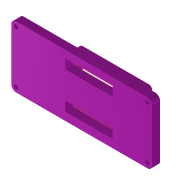
# Autodesk Inventor part: ESP32ParasiteMicroscope_base_v0
Saved by Autodesk Inventor 2022 (Build 260153000, 153)
## iProperties
Created: 2022-02-02
Part Number: ESP32ParasiteMicroscope_base_v0
Material: Generisch
Document SubType Name: Modeling
Designer: diederichbenedict
Density: 1 g/cm^3
Appearance: Glatt - Violett
Author: diederichbenedict
Autodesk Inventor part; units mm, degrees
ref_plane "YZ Plane" through (0, 0, 0) normal (1, 0, 0) x (0, 1, 0)
ref_plane "XZ Plane" through (0, 0, 0) normal (0, 1, 0) x (-1, 0, 0)
ref_plane "XY Plane" through (0, 0, 0) normal (0, 0, 1) x (1, 0, 0)
ref_plane "Arbeitsebene1" through (0, 0, 4) normal (0, 0, 1) x (1, 0, 0)
sketch "Skizze1" plane through (0, 0, 4) normal (0, 0, 1) x (1, 0, 0)
  arc A0 (-20, -12.5) -> (-19, -13.5) centre (-19, -12.5) ccw construction
  line L0 (-19, -13.5) -> (19, -13.5) construction
  arc A1 (19, -13.5) -> (20, -12.5) centre (19, -12.5) ccw construction
  line L1 (20, -12.5) -> (20, 12.5) construction
  arc A2 (20, 12.5) -> (19, 13.5) centre (19, 12.5) ccw construction
  line L2 (19, 13.5) -> (-19, 13.5) construction
  arc A3 (-19, 13.5) -> (-20, 12.5) centre (-19, 12.5) ccw construction
  line L3 (-20, 12.5) -> (-20, -12.5) construction
  line L4 (26, 12.5) -> (26, -12.5) construction
  arc A4 (19, -19.5) -> (26, -12.5) centre (19, -12.5) ccw construction
  line L5 (19, -19.5) -> (-19, -19.5) construction
  arc A5 (-26, -12.5) -> (-19, -19.5) centre (-19, -12.5) ccw construction
  line L6 (-26, -12.5) -> (-26, 12.5) construction
  arc A6 (-19, 19.5) -> (-26, 12.5) centre (-19, 12.5) ccw construction
  line L7 (-19, 19.5) -> (19, 19.5) construction
  arc A7 (26, 12.5) -> (19, 19.5) centre (19, 12.5) ccw construction
  line L8 (-24, 19.5) -> (19, 19.5)
  line L9 (19, 19.5) -> (19, -19.4749)
  line L10 (19, -19.4749) -> (-24, -19.4749)
  line L11 (-24, -19.4749) -> (-24, 19.5)
  line L12 (2.5735, 11.7657) -> (-15.3535, 11.7657) construction
  line L13 (2.5735, 13.7657) -> (-15.3535, 13.7657)
  line L14 (-15.3535, 9.7657) -> (2.5735, 9.7657)
  arc A8 (2.5735, 9.7657) -> (2.5735, 13.7657) centre (2.5735, 11.7657) ccw
  arc A9 (-15.3535, 13.7657) -> (-15.3535, 9.7657) centre (-15.3535, 11.7657) ccw
  line L15 (2.4395, -11.3613) -> (-15.3535, -11.3613) construction
  line L16 (2.4395, -9.3613) -> (-15.3535, -9.3613)
  line L17 (-15.3535, -13.3613) -> (2.4395, -13.3613)
  arc A10 (2.4395, -13.3613) -> (2.4395, -9.3613) centre (2.4395, -11.3613) ccw
  arc A11 (-15.3535, -9.3613) -> (-15.3535, -13.3613) centre (-15.3535, -11.3613) ccw
  circle A12 centre (-8.6034, 0.0126) radius 1.0539 construction
  line L18 (26.7026, 12.7126) -> (26.7026, -12.6874) construction
  line L19 (-48.7974, 12.7126) -> (26.7026, 12.7126) construction
  line L20 (-48.7974, -12.6874) -> (-48.7974, 12.7126) construction
  line L21 (26.7026, -12.6874) -> (-48.7974, -12.6874) construction
  line L22 (33.4901, -16.4749) -> (33.4901, 19.5) construction
  line L23 (30.4901, 19.5) -> (-52.5848, 19.5) construction
  line L24 (-55.5848, 19.5) -> (-55.5848, -16.4749) construction
  line L25 (-52.5848, -19.4749) -> (33.4901, -19.4749) construction
  line L26 (33.4901, 19.5) -> (19, 19.5)
  line L27 (19, 19.5) -> (19, -19.4749)
  line L28 (19, -19.4749) -> (30.4901, -19.4749)
  line L29 (33.4901, -19.4749) -> (33.4901, 16.5)
  line L30 (-24, 19.5) -> (-55.5848, 19.5)
  line L31 (-55.5848, 16.5) -> (-55.5848, -19.4749)
  line L32 (-55.5848, -19.4749) -> (-24, -19.4749)
  line L33 (-24, -19.4749) -> (-24, 19.5)
  arc A13 (-55.5848, -16.4749) -> (-52.5848, -19.4749) centre (-52.5848, -16.4749) ccw
  arc A14 (-52.5848, 19.5) -> (-55.5848, 16.5) centre (-52.5848, 16.5) ccw
  arc A15 (33.4901, 16.5) -> (30.4901, 19.5) centre (30.4901, 16.5) ccw
  arc A16 (30.4901, -19.4749) -> (33.4901, -16.4749) centre (30.4901, -16.4749) ccw
  line L34 (8.61, 8.7657) -> (-21.39, 8.7657)
  line L35 (-21.39, 8.7657) -> (-21.39, 14.7657)
  line L36 (-21.39, 14.7657) -> (8.61, 14.7657)
  line L37 (8.61, 14.7657) -> (8.61, 8.7657)
  line L38 (8.61, 8.7657) -> (-21.39, 14.7657) construction
  line L39 (-21.39, 8.7657) -> (8.61, 14.7657) construction
  line L40 (8.543, -14.3613) -> (-21.457, -14.3613)
  line L41 (-21.457, -14.3613) -> (-21.457, -8.3613)
  line L42 (-21.457, -8.3613) -> (8.543, -8.3613)
  line L43 (8.543, -8.3613) -> (8.543, -14.3613)
  line L44 (8.543, -14.3613) -> (-21.457, -8.3613) construction
  line L45 (-21.457, -14.3613) -> (8.543, -8.3613) construction
  point P0 (0, 0)
  point P1 (-15.2165, -11.3613)
  point P2 (-6.39, 11.7657)
  point P3 (-6.457, -11.3613)
  point P4 (-24, -18.4749)
  point P5 (33.4901, -16.4749)
  point P6 (30.4901, 19.5)
  point P7 (-52.5848, 19.5)
  point P8 (-55.5848, -16.4749)
  point P9 (-52.5848, -19.4749)
  dimension "d0" = 6
  dimension "d1" = 4
  dimension "d2" = 4
  dimension "d5" = 3
  dimension "d37" = 30
  dimension "d38" = 6
  dimension "d39" = 6
  dimension "d40" = 30
  constraints: 80 end point, 24 point on circle, 16 tangent, 15 parallel, 12 centre point, 9 point on line, 6 midpoint, 5 perpendicular, 4 horizontal, 3 equal radius, 14 other
  measures "d0" distance between parallel lines of L1 L4
  measures "d1" diameter of A9
  measures "d2" diameter of A11
  measures "d5" radius of A13
  measures "d37" distance of L34.start L34.end
  measures "d38" distance of L34.end L35.end
  measures "d39" distance of L40.end L41.end
  measures "d40" distance between parallel lines of L41 L43
extrude "Extrusion1" add sketch "Skizze1" along normal blind 5 contours L8 L9 L10 L11 | L11 L32 A13 L31 A14 L30 | L26 A15 L29 A16 L28 L9
sketch "Skizze3" plane through (0, 0, 4) normal (0, 0, -1) x (-1, 0, 0)
  arc A0 (-33.4901, -16.4749) -> (-30.4901, -19.4749) centre (-30.4901, -16.4749) ccw projected
  line L0 (52.5848, -19.4749) -> (-30.4901, -19.4749) projected
  arc A1 (52.5848, -19.4749) -> (55.5848, -16.4749) centre (52.5848, -16.4749) ccw projected
  line L1 (55.5848, 16.5) -> (55.5848, -16.4749) projected
  arc A2 (55.5848, 16.5) -> (52.5848, 19.5) centre (52.5848, 16.5) ccw projected
  line L2 (-30.4901, 19.5) -> (52.5848, 19.5) projected
  arc A3 (-30.4901, 19.5) -> (-33.4901, 16.5) centre (-30.4901, 16.5) ccw projected
  line L3 (-33.4901, -16.4749) -> (-33.4901, 16.5) projected
  circle A4 centre (-30.4901, 16.5) radius 1.15
  circle A5 centre (-30.4901, -16.4749) radius 1.4
  circle A6 centre (52.5848, 16.5) radius 1.4
  circle A7 centre (52.5848, -16.4749) radius 1.4
  point P0 (0, 0)
  dimension "d16" = 2.3
  dimension "d17" = 2.8
  dimension "d18" = 2.8
  dimension "d19" = 2.8
  constraints: 4 centre point, 4 coincident
  measures "d16" diameter of A4
  measures "d17" diameter of A5
  measures "d18" diameter of A6
  measures "d19" diameter of A7
extrude "Extrusion3" cut sketch "Skizze3" against normal blind 10 contours A4 | A5 | A6 | A7
sketch "Skizze9" plane through (0, 0, 4) normal (0, 0, -1) x (-1, 0, 0)
  arc A0 (19, -13.5) -> (20, -12.5) centre (19, -12.5) ccw projected
  line L0 (20, -12.5) -> (20, 12.5) projected
  arc A1 (20, 12.5) -> (19, 13.5) centre (19, 12.5) ccw projected
  line L1 (19, 13.5) -> (-19, 13.5) projected
  arc A2 (-19, 13.5) -> (-20, 12.5) centre (-19, 12.5) ccw projected
  line L2 (-20, 12.5) -> (-20, -12.5) projected
  arc A3 (-20, -12.5) -> (-19, -13.5) centre (-19, -12.5) ccw projected
  line L3 (-19, -13.5) -> (19, -13.5) projected
  line L4 (-19, 13.2) -> (19, 13.2)
  arc A4 (19.7, 12.5) -> (19, 13.2) centre (19, 12.5) ccw
  line L5 (19.7, 12.5) -> (19.7, -12.5)
  arc A5 (19, -13.2) -> (19.7, -12.5) centre (19, -12.5) ccw
  line L6 (19, -13.2) -> (-19, -13.2)
  arc A6 (-19.7, -12.5) -> (-19, -13.2) centre (-19, -12.5) ccw
  line L7 (-19.7, -12.5) -> (-19.7, 12.5)
  arc A7 (-19, 13.2) -> (-19.7, 12.5) centre (-19, 12.5) ccw
  line L8 (19, 17.2) -> (-19, 17.2)
  arc A8 (-19, 17.2) -> (-23.7, 12.5) centre (-19, 12.5) ccw
  line L9 (-23.7, 12.5) -> (-23.7, -12.5)
  arc A9 (-23.7, -12.5) -> (-19, -17.2) centre (-19, -12.5) ccw
  line L10 (-19, -17.2) -> (19, -17.2)
  arc A10 (19, -17.2) -> (23.7, -12.5) centre (19, -12.5) ccw
  line L11 (23.7, -12.5) -> (23.7, 12.5)
  arc A11 (23.7, 12.5) -> (19, 17.2) centre (19, 12.5) ccw
  point P0 (0, 0)
  dimension "d46" = 0.3
  dimension "d47" = 4
  constraints: 16 end point, 16 point on circle, 8 centre point, 14 other
  measures "d46" distance between parallel lines of L1 L4
  measures "d47" distance between parallel lines of L4 L8
ref_plane "Arbeitsebene4" through (-20, -13.5, 1.5) normal (0, 0, 1) x (1, 0, 0)
extrude "Extrusion8" add sketch "Skizze9" along normal up to surface (2.5 mm away) contours A11 L11 A10 L10 A9 L9 A8 L8
sketch "Skizze10" plane through (19, 17.2, 1.5) normal (0, 0, -1) x (-1, 0, 0)
  arc A0 (38, -30.7) -> (39, -29.7) centre (38, -29.7) ccw projected
  line L0 (39, -29.7) -> (39, -4.7) projected
  arc A1 (39, -4.7) -> (38, -3.7) centre (38, -4.7) ccw projected
  line L1 (38, -3.7) -> (0, -3.7) projected
  arc A2 (0, -3.7) -> (-1, -4.7) centre (0, -4.7) ccw projected
  line L2 (-1, -4.7) -> (-1, -29.7) projected
  arc A3 (-1, -29.7) -> (0, -30.7) centre (0, -29.7) ccw projected
  line L3 (0, -30.7) -> (38, -30.7) projected
  arc A4 (38, -30.7) -> (39, -29.7) centre (38, -29.7) ccw projected
  line L4 (38, -30.7) -> (0, -30.7) projected
  arc A5 (-1, -29.7) -> (0, -30.7) centre (0, -29.7) ccw projected
  line L5 (-1, -29.7) -> (-1, -4.7) projected
  arc A6 (0, -3.7) -> (-1, -4.7) centre (0, -4.7) ccw projected
  line L6 (0, -3.7) -> (38, -3.7) projected
  arc A7 (39, -4.7) -> (38, -3.7) centre (38, -4.7) ccw projected
  line L7 (39, -4.7) -> (39, -29.7) projected
  line L8 (38, 0) -> (0, 0) projected
  arc A8 (0, 0) -> (-4.7, -4.7) centre (0, -4.7) ccw projected
  line L9 (-4.7, -4.7) -> (-4.7, -29.7) projected
  arc A9 (-4.7, -29.7) -> (0, -34.4) centre (0, -29.7) ccw projected
  line L10 (0, -34.4) -> (38, -34.4) projected
  arc A10 (38, -34.4) -> (42.7, -29.7) centre (38, -29.7) ccw projected
  line L11 (42.7, -29.7) -> (42.7, -4.7) projected
  arc A11 (42.7, -4.7) -> (38, 0) centre (38, -4.7) ccw projected
  line L12 (0, -3.4) -> (38, -3.4)
  arc A12 (39.3, -4.7) -> (38, -3.4) centre (38, -4.7) ccw
  line L13 (39.3, -4.7) -> (39.3, -29.7)
  arc A13 (38, -31) -> (39.3, -29.7) centre (38, -29.7) ccw
  line L14 (38, -31) -> (0, -31)
  arc A14 (-1.3, -29.7) -> (0, -31) centre (0, -29.7) ccw
  line L15 (-1.3, -29.7) -> (-1.3, -4.7)
  arc A15 (0, -3.4) -> (-1.3, -4.7) centre (0, -4.7) ccw
  point P0 (19, -17.2)
  dimension "d50" = 0.3
  constraints: 8 end point, 8 point on circle, 4 centre point, 7 other
  measures "d50" distance between parallel lines of L1 L12
ref_plane "Arbeitsebene5" through (-20, -13.5, 0.5) normal (0, 0, -1) x (0, 1, 0)
extrude "Extrusion9" add sketch "Skizze10" along normal up to surface (1 mm away) contours A11 L11 A10 L10 A9 L9 A8 L8
sketch "Skizze11" plane through (19, 17.2, 0.5) normal (0, 0, -1) x (-1, 0, 0)
  arc A0 (-1.3, -29.7) -> (0, -31) centre (0, -29.7) ccw projected
  line L0 (-1.3, -4.7) -> (-1.3, -29.7) projected
  arc A1 (0, -3.4) -> (-1.3, -4.7) centre (0, -4.7) ccw projected
  line L1 (38, -3.4) -> (0, -3.4) projected
  arc A2 (39.3, -4.7) -> (38, -3.4) centre (38, -4.7) ccw projected
  line L2 (39.3, -29.7) -> (39.3, -4.7) projected
  arc A3 (38, -31) -> (39.3, -29.7) centre (38, -29.7) ccw projected
  line L3 (0, -31) -> (38, -31) projected
  line L4 (0, 0) -> (38, 0) projected
  arc A4 (0, 0) -> (-4.7, -4.7) centre (0, -4.7) ccw projected
  line L5 (-4.7, -29.7) -> (-4.7, -4.7) projected
  arc A5 (-4.7, -29.7) -> (0, -34.4) centre (0, -29.7) ccw projected
  line L6 (38, -34.4) -> (0, -34.4) projected
  arc A6 (38, -34.4) -> (42.7, -29.7) centre (38, -29.7) ccw projected
  line L7 (42.7, -4.7) -> (42.7, -29.7) projected
  arc A7 (42.7, -4.7) -> (38, 0) centre (38, -4.7) ccw projected
  line L8 (42.7, -4.7) -> (42.7, -29.7) projected
  line L9 (39.3, -29.7) -> (39.3, -4.7) projected
  line L10 (42.7, -29.7) -> (39.3, -29.7)
  line L11 (39.3, -29.7) -> (39.3, -4.7)
  line L12 (39.3, -4.7) -> (42.7, -4.7)
  line L13 (42.7, -4.7) -> (42.7, -29.7)
  line L14 (39.3, -29.7) -> (36.2612, -29.7)
  line L15 (36.2612, -29.7) -> (36.2612, -4.7)
  line L16 (36.2612, -4.7) -> (39.3, -4.7)
  line L17 (39.3, -4.7) -> (39.3, -29.7)
  point P0 (19, -17.2)
  point P1 (39.3, -4.7)
  constraints: 16 end point, 4 parallel, 2 horizontal, 2 perpendicular, 1 point on line
extrude "Extrusion10" cut sketch "Skizze11" against normal up to surface (3.5 mm away) contours L14 L15 L16 L2 | L2 L12 L7 L10
